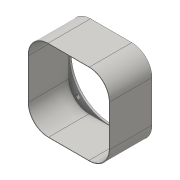
# Autodesk Inventor part: Motor mount (plain)
Saved by Autodesk Inventor 2016 (Build 200138000, 138)
## iProperties
Created: 2016-03-10
Part Number: Motor mount (plain)
Material: Generic
Document SubType Name: Modeling
Designer: s_sud
Density: 1 g/cm^3
Appearance: Default
Author: s_sud
Autodesk Inventor part; units mm, degrees
ref_plane "YZ Plane" through (0, 0, 0) normal (1, 0, 0) x (0, 1, 0)
ref_plane "XZ Plane" through (0, 0, 0) normal (0, 1, 0) x (-1, 0, 0)
ref_plane "XY Plane" through (0, 0, 0) normal (0, 0, 1) x (1, 0, 0)
sketch "Sketch1" plane through (0, 0, 0) normal (0, 1, 0) x (-1, 0, 0)
  circle A0 centre (0, 0) radius 39.5
  circle A1 centre (0, 0) radius 40.5
  dimension "d0" = 79
  dimension "d1" = 81
  constraints: 2 centre point, 2 coincident
  measures "d0" diameter of A0
  measures "d1" diameter of A1
extrude "Extrusion1" add sketch "Sketch1" along normal blind 2
sketch "Sketch21" plane through (0, 2, 0) normal (0, 1, 0) x (1, 0, 0)
  line L0 (-40.5, -40.5) -> (40.5, -40.5)
  line L1 (40.5, -40.5) -> (40.5, 40.5)
  line L2 (40.5, 40.5) -> (-40.5, 40.5)
  line L3 (-40.5, 40.5) -> (-40.5, -40.5)
  line L4 (-40.5, -40.5) -> (40.5, 40.5) construction
  line L5 (40.5, -40.5) -> (-40.5, 40.5) construction
  circle A0 centre (0, 0) radius 40.5
  dimension "d111" = 81
  dimension "d112" = 81
  constraints: 12 end point, 2 midpoint, 2 parallel, 1 centre point, 1 coincident, 1 horizontal, 1 perpendicular, 1 tangent
  measures "d111" distance of L2.end L0.start
  measures "d112" distance of L0.start L0.end
extrude "Extrusion21" add sketch "Sketch21" against normal blind 2 contours L3 A0 L0 | A0 L1 L0 | L3 L2 A0 | A0 L2 L1
fillet "Fillet3" radius 20 4 edges at (-40.5, 1, -40.5) (40.5, 1, -40.5) (40.5, 1, 40.5) (-40.5, 1, 40.5)
sketch "Sketch24" plane through (0, 0, 0) normal (0, -1, 0) x (1, 0, 0)
  arc A0 (-20.5, 40.5) -> (-40.5, 20.5) centre (-20.5, 20.5) ccw projected
  circle A1 centre (0, 0) radius 39.5 projected
  arc A2 (-20.5, 40.5) -> (-40.5, 20.5) centre (-20.5, 20.5) ccw projected
  line L0 (-40.5, 20.5) -> (-40.5, -20.5) projected
  arc A3 (-40.5, -20.5) -> (-20.5, -40.5) centre (-20.5, -20.5) ccw projected
  line L1 (-20.5, -40.5) -> (20.5, -40.5) projected
  arc A4 (20.5, -40.5) -> (40.5, -20.5) centre (20.5, -20.5) ccw projected
  line L2 (40.5, -20.5) -> (40.5, 20.5) projected
  arc A5 (40.5, 20.5) -> (20.5, 40.5) centre (20.5, 20.5) ccw projected
  line L3 (20.5, 40.5) -> (-20.5, 40.5) projected
  line L4 (-20, -40) -> (20, -40)
  line L5 (40, -20) -> (40, 20)
  line L6 (20, 40) -> (-20, 40)
  line L7 (-40, 20) -> (-40, -20)
  line L8 (-40, -40) -> (40, 40) construction
  line L9 (40, -40) -> (-40, 40) construction
  arc A6 (-38, 40) -> (-40, 38) centre (-38, 38) ccw
  arc A7 (40, 20) -> (20, 40) centre (20, 20) ccw
  arc A8 (-20, 40) -> (-40, 20) centre (-20, 20) ccw
  arc A9 (-40, -20) -> (-20, -40) centre (-20, -20) ccw
  arc A10 (20, -40) -> (40, -20) centre (20, -20) ccw
  dimension "d133" = 80
  dimension "d134" = 80
  dimension "d135" = 2
  dimension "d136" = 20
  constraints: 12 end point, 10 point on circle, 10 point on line, 10 tangent, 5 centre point, 3 equal radius, 2 midpoint, 2 parallel, 1 horizontal, 1 perpendicular
  measures "d133" distance of L9.end L8.end
  measures "d134" distance of L9.start L8.end
  measures "d135" radius of A6
  measures "d136" radius of A7
extrude "Extrusion24" add sketch "Sketch24" along normal blind 40 contours L3 A5 L2 A4 L1 A3 L0 A0
sketch "Sketch25" plane through (0, 0, 0) normal (0, -1, 0) x (1, 0, 0)
  circle A0 centre (-31, -31) radius 2
  line L0 (0, 0) -> (-40.0942, -40.0942)
  line L1 (0, 0) -> (0, -34.7078)
  circle A1 centre (31, -31) radius 2
  circle A2 centre (31, 31) radius 2
  circle A3 centre (-31, 31) radius 2
  dimension "d139" = 4
  dimension "d140" = 31
  dimension "d141" = 45
  dimension "d144" = 360
  constraints: 4 centre point, 4 end point, 1 point on line, 1 vertical, 9 other
  measures "d139" diameter of A0
  measures "d140" horizontal distance of L0.start A0.centre
  measures "d141" angle of L1 L0
extrude "Extrusion25" cut sketch "Sketch25" against normal blind 10
body "Solid1"
